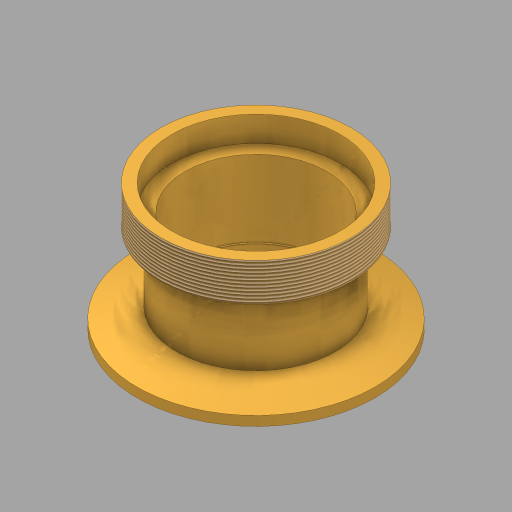
# Autodesk Inventor part: KF_fitting
Saved by Autodesk Inventor 2024 (Build 280153020, 153B)
## iProperties
Created: 2023-11-04
Part Number: KF_fitting
Material: Brass, Soft Yellow
Document SubType Name: Modeling
Designer: schanen
Density: 8.47 g/cm^3
Appearance: Brass - Satin
Mass: 269.733 g
Surface Area: 196.65 cm^2
Volume: 31.8456 cm^3
neck_thread_dia: 30.000 mm
neck_thread_len: 12.000 mm
neck_ir: 22.325 mm
Author: schanen
Autodesk Inventor part; units mm, degrees
ref_plane "YZ Plane" through (0, 0, 0) normal (1, 0, 0) x (0, 1, 0)
ref_plane "XZ Plane" through (0, 0, 0) normal (0, 1, 0) x (-1, 0, 0)
ref_plane "XY Plane" through (0, 0, 0) normal (0, 0, 1) x (1, 0, 0)
sketch "Sketch1" plane through (0, 0, 0) normal (0, 0, 1) x (1, 0, 0)
  line L0 (-22.325, 24) -> (-22.325, 0)
  line L1 (-25, -1.6506) -> (-25, 20)
  line L2 (-25, 20) -> (-30, 20)
  line L3 (-30, 20) -> (-30, 32)
  line L4 (-30, 32) -> (-26.5, 32)
  line L5 (-26.5, 32) -> (-26.5, 24)
  line L6 (-26.5, 24) -> (-22.325, 24)
  line L7 (0, -16) -> (0, 40) projected
  line L8 (-25, -1.6506) -> (-37.5, -5)
  line L9 (-37.5, -5) -> (-37.5, -8)
  line L10 (-37.5, -8) -> (-26, -8)
  line L11 (-26, -8) -> (-26, -5)
  line L12 (-26, -5) -> (-21.75, -5)
  line L13 (-21.75, -5) -> (-21.75, 0)
  line L14 (-21.75, 0) -> (-22.325, 0)
  point P0 (0, 0)
  dimension "neck_ir" = 22.325
  dimension "d4" = 8
  dimension "neck_thread_dia" = 30
  dimension "neck_thread_len" = 12
  dimension "d14" = 26
  dimension "d15" = 21.75
  dimension "d16" = 3
  dimension "d17" = 15
  dimension "d18" = 3
  dimension "d19" = 37.5
  dimension "d20" = 25
  dimension "d22" = 5
  dimension "d23" = 26.5
  dimension "d24" = 40
  constraints: 28 end point, 9 perpendicular, 2 vertical, 1 horizontal, 1 horizontal alignment
  measures "neck_ir" distance from line of point (0, 0) L0
  measures "d4" distance of L4.end L5.end
  measures "neck_thread_dia" distance from line of point (0, 0) L3
  measures "neck_thread_len" distance of L2.end L3.end
  measures "d14" distance between parallel lines of L7 L11
  measures "d15" distance between parallel lines of L7 L13
  measures "d16" distance of L8.end L9.end
  measures "d17" angle of L8 L10
  measures "d18" distance of L10.end L11.end
  measures "d19" distance between parallel lines of L7 L9
  measures "d20" distance between parallel lines of L7 L1
  measures "d22" distance of L12.end L13.end
  measures "d23" distance between parallel lines of L7 L5
  measures "d24" vertical distance of L9.end L3.end
revolve "Revolution1" add sketch "Sketch1" angle 360 about axis through (0, -10, 0) along (0, 1, 0)
thread "Thread1" size "M60x1" class "6g" standard "ANSI Metric M Profile" full length
equation "\"d4\" = 2 * oring_dia"
equation "\"d23\" = 0.5 * oring_od"
equation "\"oring_diameter\" = 4"
equation "\"oring_dia\" = 4"
equation "\"oring_od\" = 53"
body "Solid1"
